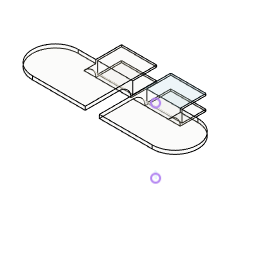
Desk Attached Mousepad v2 (Autodesk Fusion 360 design; units mm, degrees)
Autodesk Fusion 360 part; units mm, degrees
sketch "Sketch1" plane through (0, 0, 0) normal (0, 1, 0) x (1, 0, 0)
  line L0 (2.9948, -0.9169) -> (7.4948, -0.9169)
  line L1 (7.4948, -0.9169) -> (7.4948, -18.9169)
  line L2 (7.4948, -18.9169) -> (2.9948, -18.9169)
  line L3 (2.9948, -18.9169) -> (2.9948, -0.9169)
  dimension "d1" = 4.5
  dimension "d2" = 18
  constraint horizontal L0
  constraint vertical L1
  constraint horizontal L2
  constraint vertical L3
  measures "d1" distance of L0.start L0.end
  measures "d2" distance of L0.start L2.end
sketch "Sketch2" plane through (0, 0, 18.9169) normal (0, 0, 1) x (-1, 0, 0)
  line L0 (-2.9948, 0) -> (-7.4948, 0)
  line L1 (-7.4948, 0) -> (-7.4948, -2)
  line L2 (-7.4948, -2) -> (-2.9948, -2)
  line L3 (-2.9948, -2) -> (-2.9948, 0)
  line L4 (-7.4948, 0) -> (-2.9948, 0)
  line L5 (-2.9948, 0.5) -> (-7.4948, 0.5)
  line L6 (-2.9948, 0) -> (-3.4948, 0)
  line L7 (-3.4948, -2) -> (-2.9948, -2)
  line L8 (-2.9948, -2) -> (-2.9948, 0)
  line L9 (-2.9948, -2) -> (-7.4948, -2)
  line L10 (-7.4948, -2.5) -> (-2.9948, -2.5)
  line L11 (-7.4948, 0.5) -> (-7.9948, 0.5)
  line L12 (-7.9948, 0.5) -> (-7.9948, -2.5)
  line L13 (-7.9948, -2.5) -> (-7.4948, -2.5)
  line L14 (-2.9948, 0.5) -> (-2.4948, 0.5)
  line L15 (-2.4948, 0.5) -> (-2.4948, -2.5)
  line L16 (-2.4948, -2.5) -> (-2.9948, -2.5)
  dimension "d5" = 0.5
  dimension "d6" = 0.5
  dimension "d7" = 2
  dimension "d8" = 4.5
  dimension "d9" = 0.5
  dimension "d10" = 0.5
  dimension "d11" = 3
  dimension "d12" = 0.5
  dimension "d13" = 3
  constraint horizontal L4
  constraint horizontal L5
  constraint coincident L0.end L1.start
  constraint horizontal L6
  constraint horizontal L7
  constraint vertical L8
  constraint coincident L0.start L3.end
  constraint horizontal L9
  constraint horizontal L10
  constraint coincident L2.end L3.start
  constraint horizontal L11
  constraint vertical L12
  constraint horizontal L13
  constraint horizontal L14
  constraint vertical L15
  constraint horizontal L16
  measures "d5" distance of L0.end L5.end
  measures "d6" distance of L0.start L6.end
  measures "d7" distance of L0.start L2.end
  measures "d8" distance of L2.end L1.end
  measures "d9" distance of L2.end L10.end
  measures "d10" distance of L5.end L11.end
  measures "d11" distance of L5.end L10.start
  measures "d12" distance of L5.start L14.end
  measures "d13" distance of L5.start L10.end
extrude "Extrude2" add sketch "Sketch2" against normal blind 18 makes body 1
sketch "Sketch3" plane through (0, 0, 0.9169) normal (0, 0, -1) x (1, 0, 0)
  line L0 (2.9948, 0) -> (7.4948, 0)
  line L1 (7.4948, 0) -> (7.4948, -2)
  line L2 (7.4948, -2) -> (2.9948, -2)
  line L3 (2.9948, -2) -> (2.9948, 0)
  line L4 (7.9948, 0.5) -> (2.4948, 0.5)
  line L5 (2.4948, 0.5) -> (2.4948, -2.5)
  line L6 (2.4948, -2.5) -> (7.9948, -2.5)
  line L7 (7.9948, -2.5) -> (7.9948, 0.5)
  line L8 (7.9948, 0.5) -> (2.4948, 0.5)
  line L9 (2.4948, 0.5) -> (2.4948, -2.5)
  line L10 (2.4948, -2.5) -> (7.9948, -2.5)
  line L11 (7.9948, -2.5) -> (7.9948, 0.5)
  constraint horizontal L8
  constraint vertical L9
  constraint horizontal L10
  constraint vertical L11
  constraint coincident L5.end L6.start
  constraint coincident L4.start L7.end
extrude "Extrude3" add sketch "Sketch3" along normal blind 0.5 contours L0 L1 L2 L3 | L4 L5 L6 L7 L8 L9 L10 L11 bodies 1
sketch "Sketch4" plane through (0, 2.5, 0) normal (0, 1, 0) x (-1, 0, 0)
  line L0 (-2.4948, 18.9169) -> (-7.9948, 18.9169)
  line L1 (-7.9948, 18.9169) -> (-7.9948, 0.4169)
  line L2 (-7.9948, 0.4169) -> (-2.4948, 0.4169)
  line L3 (-2.4948, 0.4169) -> (-2.4948, 18.9169)
scale "Scale1" factor 10 about (7.9948, -0.5, 18.9169) bodies 1
sketch "Sketch5" plane through (0, 29.5, 0) normal (0, 1, 0) x (-1, 0, 0)
  line L0 (47.0052, 18.9169) -> (-7.9948, 18.9169)
  line L1 (-7.9948, 18.9169) -> (-7.9948, -166.0831)
  line L2 (-7.9948, -166.0831) -> (47.0052, -166.0831)
  line L3 (47.0052, -166.0831) -> (47.0052, 18.9169)
  line L4 (-7.9948, 18.9169) -> (47.0052, 18.9169)
  line L5 (47.0052, 18.9169) -> (47.0052, 13.9169)
  line L6 (47.0052, 13.9169) -> (-7.9948, 13.9169)
  line L7 (-7.9948, 13.9169) -> (-7.9948, 18.9169)
  line L8 (-7.9948, -20.0831) -> (47.0052, -20.0831)
  line L9 (47.0052, -20.0831) -> (47.0052, -25.0831)
  line L10 (47.0052, -25.0831) -> (-7.9948, -25.0831)
  line L11 (-7.9948, -25.0831) -> (-7.9948, -20.0831)
  dimension "d19" = 5
  dimension "d20" = 34
  dimension "d21" = 5
  constraint horizontal L4
  constraint vertical L5
  constraint horizontal L6
  constraint vertical L7
  constraint coincident L0.end L1.start
  constraint horizontal L8
  constraint vertical L9
  constraint horizontal L10
  constraint vertical L11
  measures "d19" distance of L0.end L6.end
  measures "d20" distance of L6.end L8.start
  measures "d21" distance of L8.start L10.end
extrude "Extrude4" add sketch "Sketch5" along normal blind 65 contours L0 L1 L3 L4 L5 L6 L7 | L1 L3 L8 L9 L10 L11 bodies 1
move_body "Move1" bodies 1 to x (1, 0, 0) y (0, 1, 0) z (0, 0, 1) at (0, 0, 170)
sketch "Sketch6" plane through (7.9948, 0, 0) normal (1, 0, 0) x (0, 1, 0)
  line L0 (94.5, 188.9169) -> (-0.5, 188.9169)
  line L1 (-0.5, 3.9169) -> (29.5, 3.9169)
  line L2 (29.5, 3.9169) -> (29.5, 144.9169)
  line L3 (29.5, 144.9169) -> (94.5, 144.9169)
  line L4 (94.5, 144.9169) -> (94.5, 149.9169)
  line L5 (94.5, 149.9169) -> (29.5, 149.9169)
  line L6 (29.5, 149.9169) -> (29.5, 183.9169)
  line L7 (29.5, 183.9169) -> (94.5, 183.9169)
  line L8 (94.5, 183.9169) -> (94.5, 188.9169)
sketch "Sketch7" plane through (-47.0052, 0, 0) normal (-1, 0, 0) x (0, -1, 0)
  line L0 (0.5, 188.9169) -> (-94.5, 188.9169)
  line L1 (-94.5, 188.9169) -> (-94.5, 183.9169)
  line L2 (-94.5, 183.9169) -> (-29.5, 183.9169)
  line L3 (-29.5, 183.9169) -> (-29.5, 149.9169)
  line L4 (-29.5, 149.9169) -> (-94.5, 149.9169)
  line L5 (-94.5, 149.9169) -> (-94.5, 144.9169)
  line L6 (-94.5, 144.9169) -> (-29.5, 144.9169)
  line L7 (-29.5, 144.9169) -> (-29.5, 3.9169)
  line L8 (-29.5, 3.9169) -> (0.5, 3.9169)
  line L9 (0.5, 3.9169) -> (0.5, 188.9169)
extrude "Extrude5" cut 2 faces at (-10.3385, 29.5, 172.5836) (-10.3385, 29.5, 50.9169) along direction (0, -1, 0) blind 3 on bodies 1 bodies 1
extrude "Extrude6" cut 1 faces at (-10.3385, -0.5, 127.2503) along direction (0, 1, 0) blind 3 on bodies 1 bodies 1
extrude "Extrude7" cut sketch "Sketch7" against normal blind 3 bodies 1
extrude "Extrude8" cut 1 faces at (7.9948, 10.5, 112.5836) along direction (-1, 0, 0) blind 3 on bodies 1 bodies 1
split "Split1" by plane through (-47.0052, 29.5, 144.9169) normal (0, 0, -1) bodies 1 makes body 2 at (-27.6718, 26.5, 97.9169)
delete_body "RemoveBody1" bodies 2
split "Split2" by plane through (2.9948, 24.5, 188.9169) normal (0, -1, 0) bodies 1 makes body 3 at (-11.3385, 2.5, 174.2503)
delete_body "RemoveBody2" bodies 3
extrude "Extrude9" add 3 faces at (3.6615, 24.5, 174.2503) (-12.0052, 24.5, 174.2503) (-42.6718, 24.5, 174.2503) along direction (0, -1, 0) blind 3 on bodies 1 bodies 1
move_face "OffsetFaces1" offset 1 1 faces at (4.9948, 47.5, 187.2503) on bodies 1
extrude "Extrude10" add 1 faces at (5.9948, 47.5, 187.2503) along direction (1, 0, 0) blind 50 on bodies 1 bodies 1
sketch "Sketch8" plane through (0, 0, 188.9169) normal (0, 0, 1) x (-1, 0, 0)
  line L0 (-55.9948, -94.5) -> (44.0052, -94.5)
  line L1 (44.0052, -94.5) -> (44.0052, -21.5)
  line L2 (44.0052, -21.5) -> (-55.9948, -21.5)
  line L3 (-55.9948, -21.5) -> (-55.9948, -94.5)
sketch "Sketch9" plane through (0, 0, 188.9169) normal (0, 0, 1) x (-1, 0, 0)
copy_body "CopyPasteBodies1" bodies 1 makes body 4
move_body "Move2" bodies 4 to x (1, 0, 0) y (0, 1, 0) z (0, 0, 1) at (-140, 0, 0)
sketch "Sketch10" plane through (0, 0, 188.9169) normal (0, 0, 1) x (-1, 0, 0)
  line L0 (84.0052, -94.5) -> (184.0052, -94.5)
  line L1 (184.0052, -94.5) -> (184.0052, -21.5)
  line L2 (184.0052, -21.5) -> (84.0052, -21.5)
  line L3 (84.0052, -21.5) -> (84.0052, -94.5)
  line L4 (84.0052, -21.5) -> (234.0052, -21.5)
  line L5 (234.0052, 108.5) -> (84.0052, 108.5)
  line L6 (84.0052, 108.5) -> (84.0052, -21.5)
  arc A0 (234.0052, -21.5) -> (234.0052, 108.5) centre (234.0052, 43.5) ccw
  dimension "d39" = 150
  dimension "d40" = 130
  constraint horizontal L4
  constraint horizontal L5
  constraint vertical L6
  constraint coincident L2.end L3.start
  constraint tangent L4 A0
  measures "d39" distance of L2.end L4.end
  measures "d40" distance of L2.end L5.end
sketch "Sketch11" plane through (0, 0, 188.9169) normal (0, 0, 1) x (1, 0, 0)
sketch "Sketch12" plane through (0, 0, 188.9169) normal (0, 0, 1) x (1, 0, 0)
sketch "Sketch13" plane through (0, 0, 188.9169) normal (0, 0, 1) x (1, 0, 0)
sketch "Sketch14" plane through (0, 0, 188.9169) normal (0, 0, 1) x (-1, 0, 0)
sketch "Sketch15" plane through (0, 0, 188.9169) normal (0, 0, 1) x (1, 0, 0)
sketch "Sketch16" plane through (0, 0, 188.9169) normal (0, 0, 1) x (-1, 0, 0)
  line L0 (44.0052, -21.5) -> (-105.9948, -21.5)
  line L1 (-105.9948, 108.5) -> (44.0052, 108.5)
  line L2 (44.0052, 108.5) -> (44.0052, -21.5)
  arc A0 (-105.9948, 108.5) -> (-105.9948, -21.5) centre (-105.9948, 43.5) ccw
  point P0 (44.0052, -21.5)
  dimension "d42" = 150
  dimension "d43" = 130
  constraint horizontal L0
  constraint horizontal L1
  constraint vertical L2
  constraint coincident P0 L0.start
  constraint tangent L0 A0
  measures "d42" distance of P0 L0.end
  measures "d43" distance of P0 L1.end
extrude "Extrude11" add sketch "Sketch10" sketch "Sketch16" against normal blind 10 contours L2 L4 L5 L6 A0 of sketch 2 bodies 1 4
fillet "Fillet1" radius 34 1 edges at (-134.0052, 21.5, 178.9169) on bodies 4
fillet "Fillet2" radius 34 1 edges at (5.9948, 21.5, 178.9169) on bodies 1
